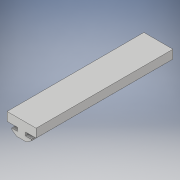
# Autodesk Inventor part: Sliderfor2020
Saved by Autodesk Inventor 2017 (Build 210142000, 142)
## iProperties
Created: 2017-12-08
Part Number: Sliderfor2020
Material: Generic
Document SubType Name: Modeling
Designer: User
Density: 1 g/cm^3
Appearance: Default
Author: User
Autodesk Inventor part; units mm, degrees
ref_plane "YZ Plane" through (0, 0, 0) normal (1, 0, 0) x (0, 1, 0)
ref_plane "XZ Plane" through (0, 0, 0) normal (0, 1, 0) x (-1, 0, 0)
ref_plane "XY Plane" through (0, 0, 0) normal (0, 0, 1) x (1, 0, 0)
sketch "Sketch1" plane through (0, 0, 0) normal (0, 0, 1) x (1, 0, 0)
  line L0 (0, 0) -> (14.5304, 0)
  line L1 (-8.7854, 6.6412) -> (8.2146, 6.6412)
  line L2 (8.2146, 6.6412) -> (8.2146, 1.6412)
  line L3 (8.2146, 1.6412) -> (2.0946, 1.6412)
  line L4 (2.0946, 1.6412) -> (2.0946, -0.3588)
  line L5 (2.0946, -0.3588) -> (5.4596, -0.3588)
  line L6 (2.5721, -3.1588) -> (-3.1429, -3.1588)
  line L7 (-3.1429, -3.1588) -> (-6.0304, -1.1208)
  line L8 (-6.0304, -1.1208) -> (-6.0304, -0.3588)
  line L9 (-6.0304, -0.3588) -> (-2.6654, -0.3588)
  line L10 (-2.6654, -0.3588) -> (-2.6654, 1.6412)
  line L11 (-2.6654, 1.6412) -> (-8.7854, 1.6412)
  line L12 (-8.7854, 1.6412) -> (-8.7854, 6.6412)
  line L13 (5.4596, -0.3588) -> (5.4596, -1.1208)
  line L14 (5.4596, -1.1208) -> (2.5721, -3.1588)
  dimension "d0" = 17
  dimension "d1" = 9.8
  dimension "d2" = 5
  dimension "d3" = 2
  dimension "d4" = 4.76
  dimension "d6" = 11.49
  dimension "d7" = 2.755
  dimension "d8" = 5.715
  dimension "d9" = 5.6425
  dimension "d10" = 6.12
  dimension "d11" = 0.762
  dimension "d12" = 0.762
  constraints: 30 end point, 7 perpendicular, 4 point on line, 2 horizontal, 1 vertical
  measures "d0" distance of L1.start L1.end
  measures "d1" vertical distance of L6.end L1.start
  measures "d2" distance between parallel lines of L11 L1
  measures "d3" distance between parallel lines of L9 L11
  measures "d4" distance between parallel lines of L4 L10
  measures "d6" distance between parallel lines of L8 L13
  measures "d7" distance between parallel lines of L8 L12
  measures "d8" distance of L6.start L6.end
  measures "d9" distance from line of L6.end L12
  measures "d10" distance between parallel lines of L12 L10
  measures "d11" distance of L7.end L8.end
  measures "d12" distance of L5.end L13.end
extrude "Extrusion1" add sketch "Sketch1" along normal blind 80
equation "\"d7\" = -0.5 * d6 + 0.5 * d0"
equation "\"d9\" = -0.5 * d8 + 0.5 * d0"
equation "\"d10\" = -0.5 * d4 + 0.5 * d0"
equation "\"d12\" = d11"
body "Solid1"
